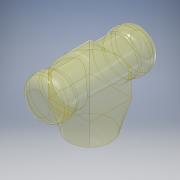
# Autodesk Inventor part: Palu
Saved by Autodesk Inventor 2017 (Build 210142000, 142)
## iProperties
Created: 2021-02-25
Part Number: Palu
Material: Generic
Document SubType Name: Modeling
Designer: Lenovo Y900
Density: 1 g/cm^3
Appearance: Clear - Yellow
Author: Lenovo Y900
Autodesk Inventor part; units mm, degrees
sketch "Sketch2" plane through (0, 0, 0) normal (0, 0, 1) x (1, 0, 0)
  circle A0 centre (0, 0) radius 7.5
  dimension "d1" = 15
  constraints: 1 centre point, 1 coincident
  measures "d1" diameter of A0
ref_plane "Work Plane1" through (0, 0, 10) normal (0, 0, 1) x (1, 0, 0)
sketch "Sketch3" plane through (0, 0, 10) normal (0, 0, 1) x (1, 0, 0)
  line L0 (-7.5, -7.5) -> (7.5, -7.5)
  line L1 (7.5, -7.5) -> (7.5, 7.5)
  line L2 (7.5, 7.5) -> (-7.5, 7.5)
  line L3 (-7.5, 7.5) -> (-7.5, -7.5)
  line L4 (-7.5, -7.5) -> (7.5, 7.5) construction
  line L5 (7.5, -7.5) -> (-7.5, 7.5) construction
  point P0 (0, 0)
  dimension "d5" = 15
  dimension "d6" = 15
  constraints: 12 end point, 2 midpoint, 2 parallel, 1 horizontal, 1 perpendicular
  measures "d5" distance of L2.end L1.end
  measures "d6" distance of L1.end L0.end
loft "Loft1" add profiles "Sketch2", "Sketch3"
sketch "Sketch4" plane through (-7.5, -7.5, 10) normal (0, 0, 1) x (1, 0, 0)
  line L0 (12.8033, 12.8033) -> (15, 15) projected
  line L1 (0, 0) -> (15, 0)
  line L2 (15, 0) -> (15, 15)
  line L3 (15, 15) -> (0, 15)
  line L4 (0, 15) -> (0, 0)
  line L5 (0, 0) -> (15, 15) construction
  line L6 (15, 0) -> (0, 15) construction
  point P0 (7.5, 7.5)
  dimension "d11" = 15
  dimension "d12" = 15
  constraints: 12 end point, 2 midpoint, 2 parallel, 1 horizontal, 1 perpendicular
  measures "d11" distance of L3.end L0.end
  measures "d12" distance of L0.end L1.end
extrude "Extrusion2" add sketch "Sketch4" along normal blind 15
sketch "Sketch5" plane through (-7.5, -7.5, 25) normal (0, -1, 0) x (1, 0, 0)
  circle A0 centre (7.5, -7.5) radius 6.5
  point P0 (7.5, -25)
  point P1 (15, -15)
  dimension "d15" = 13
  constraints: 1 centre point, 1 coincident
  measures "d15" diameter of A0
extrude "Extrusion3" add sketch "Sketch5" along normal blind 5
sketch "Sketch6" plane through (0, -12.5, 17.5) normal (0, -1, 0) x (1, 0, 0)
  circle A0 centre (0, 0) radius 7.5
  point P0 (0, -17.5)
  dimension "d24" = 15
  constraints: 1 centre point
  measures "d24" diameter of A0
ref_plane "Work Plane2" through (0, -18.5, 17.5) normal (0, -1, 0) x (1, 0, 0)
sketch "Sketch7" plane through (0, -18.5, 17.5) normal (0, -1, 0) x (1, 0, 0)
  circle A0 centre (0, 0) radius 6.5
  point P0 (0, -17.5)
  constraints: 1 centre point
loft "Loft2" add profiles "Sketch6", "Sketch7"
fillet "Fillet1" radius 2 1 edges at (-6.5, -12.5, 17.5)
fillet "Fillet2" radius 3 1 edges at (-6.5, -18.5, 17.5)
fillet "Fillet3" radius 5 1 edges at (-7.5, -12.5, 17.5)
ref_plane "Work Plane3" through (-7.5, 0, 25) normal (0, -1, 0) x (1, 0, 0)
mirror "Mirror1" about plane through (-7.5, 0, 25) normal (0, -1, 0) of "Fillet2", "Loft2", "Fillet3", "Fillet1", "Extrusion3"
fillet "Fillet4" radius 7.25 4 edges at (-7.5, 0, 25) (0, 7.5, 25) (7.5, 0, 25) (0, -7.5, 25)
body "Solid2"
